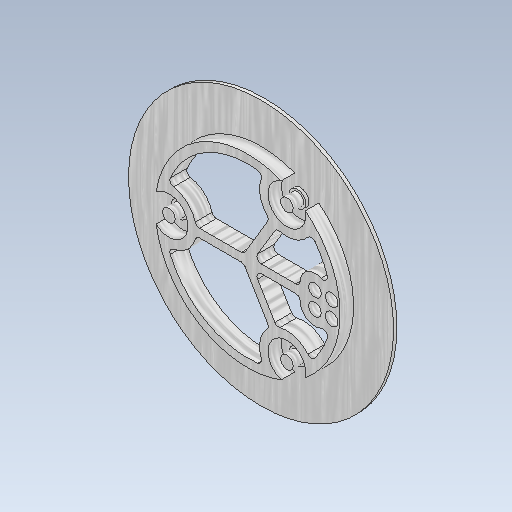
# Autodesk Inventor part: クランク4t
Saved by Autodesk Inventor 2020.2 (Build 242310000, 310)
## iProperties
Created: 2020-04-13
Part Number: クランク4t
Material: アルミニウム 7075
Document SubType Name: Modeling
Designer: aoyama
Density: 2.81 g/cm^3
Appearance: サテン - ブラシ仕上げ 重厚
Author: aoyama
Autodesk Inventor part; units mm, degrees
ref_plane "YZ Plane" through (0, 0, 0) normal (1, 0, 0) x (0, 1, 0)
ref_plane "XZ Plane" through (0, 0, 0) normal (0, 1, 0) x (-1, 0, 0)
ref_plane "XY Plane" through (0, 0, 0) normal (0, 0, 1) x (1, 0, 0)
sketch "スケッチ1" plane through (0, 0, 0) normal (0, 0, 1) x (1, 0, 0)
  circle A0 centre (-18, 0) radius 31.5
  line L0 (0, 0) -> (-18, 0) construction
  circle A1 centre (-36.7, 0) radius 1.5
  circle A2 centre (-36.7, 0) radius 4 construction
  circle A3 centre (-36.7, 0) radius 4.5
  circle A4 centre (-8.65, -16.1947) radius 4.5
  circle A5 centre (-8.65, -16.1947) radius 4 construction
  circle A6 centre (-8.65, -16.1947) radius 1.5
  circle A7 centre (-8.65, 16.1947) radius 4.5
  circle A8 centre (-8.65, 16.1947) radius 4 construction
  circle A9 centre (-8.65, 16.1947) radius 1.5
  circle A10 centre (-18, 0) radius 22
  line L1 (-36.7, 0) -> (-18, 0) construction
  circle A11 centre (-18, 0) radius 22.7 construction
  circle A12 centre (-36.7, 0) radius 2
  circle A13 centre (-8.65, -16.1947) radius 2
  circle A14 centre (-8.65, 16.1947) radius 2
  circle A15 centre (-1.9799, 1.9799) radius 2.8
  circle A16 centre (-1.9799, 1.9799) radius 1.5
  circle A17 centre (-1.9799, -1.9799) radius 1.5
  circle A18 centre (-1.9799, -1.9799) radius 2.8
  circle A19 centre (1.9799, -1.9799) radius 1.5
  circle A20 centre (1.9799, -1.9799) radius 2.8
  circle A21 centre (1.9799, 1.9799) radius 1.5
  circle A22 centre (1.9799, 1.9799) radius 2.8
  line L2 (0, 0) -> (-1.9799, 1.9799)
  point P0 (-1.5877, 1.6905)
  point P1 (-5.0591, 12.5113)
  point P2 (1.2886, 2.8639)
  point P3 (1.2886, -2.8639)
  point P4 (-5.0591, -12.5113)
  point P5 (-13.6354, -17.4628)
  point P6 (-35.3056, -4.9515)
  point P7 (-35.3056, 4.9515)
  point P8 (-13.6354, 17.4628)
  point P9 (0.5827, -2.75)
  point P10 (-4.16, 16.8432)
  point P11 (-4.16, -16.8432)
  point P12 (-10.3333, -20.4074)
  point P13 (-39.5067, -3.5642)
  point P14 (-39.5067, 3.5642)
  point P15 (-10.3333, 20.4074)
  point P16 (-0.2113, 2.75)
  point P17 (-35.9375, 1.4987)
  point P18 (-35.9375, -1.4987)
  point P19 (-7.7333, -14.785)
  point P20 (-10.3292, -16.2837)
  point P21 (-10.3292, 16.2837)
  point P22 (-7.7333, 14.785)
  point P23 (4, 0.041)
  point P24 (4, -0.041)
  point P25 (3.5801, -4.2776)
  point P26 (-4.2595, -17.1813)
  point P27 (-9.9908, -20.4903)
  point P28 (-39.7497, -3.3089)
  point P29 (-39.7497, 3.3089)
  point P30 (-9.9908, 20.4903)
  point P31 (-4.2595, 17.1813)
  point P32 (3.5801, 4.2776)
  dimension "d10" = 63
  dimension "d13" = 3
  dimension "d14" = 8
  dimension "d15" = 9
  dimension "d16" = 360
  dimension "d19" = 9.5
  dimension "d23" = 4
  dimension "d24" = 360
  dimension "d25" = 5.6
  dimension "d26" = 3
  dimension "d30" = 360
  dimension "d46" = 45
  dimension "d47" = 18
  dimension "d49" = 44
  dimension "d50" = 18.7
  dimension "d53" = 0.7
  dimension "d69" = 45.4
  constraints: 23 centre point, 15 coincident, 6 end point, 2 horizontal, 2 tangent, 44 other
  measures "d10" diameter of A0
  measures "d13" diameter of A1
  measures "d14" diameter of A2
  measures "d15" diameter of A3
  measures "d19" radial gap between concentric circles of A10 A0
  measures "d23" diameter of A12
  measures "d25" diameter of A15
  measures "d26" diameter of A16
  measures "d46" angle of L0 L2
  measures "d47" distance of L0.end point (0, 0)
  measures "d49" diameter of A10
  measures "d50" distance of A0.centre A14.centre
  measures "d53" radial gap between concentric circles of A10 A11
  measures "d69" diameter of A11
extrude "押し出し1" add sketch "スケッチ1" along normal blind 0.8 contours A0 | A3 A10 | A10 A3 | A10 A7 | A7 A10 | A10 A4 | A4 A10 | A22 A10 | A10 A20
extrude "押し出し2" add sketch "スケッチ1" along normal blind 1.5 contours A12 | A13 | A14
extrude "押し出し3" add sketch "スケッチ1" along normal blind 4 contours A1 | A3 A10 A7 A22 A15 A18 A20 A4 | A10 A22 A20 A21 A15 | A20 A18 A19 A22 A10 | A10 A20 A22 | A22 A16 A18 A15 | A15 A21 A22 A16 | A20 A17 A18 A19 | A18 A15 A17 A20 | A22 A19 A20 A21 | A18 A16 A15 A17 | A21 A20 A15 | A22 L2 A16 | A18 A22 A19 | A17 A15 A20 | A18 A16 L2 | A6 | A9 picked at (0.5491, 0.5309) picked at (0.5491, -0.5309) picked at (-0.5491, -0.5309)
sketch "スケッチ2" plane through (0, 0, 4) normal (0, 0, 1) x (1, 0, 0)
  arc A0 (-39.7497, -3.3089) -> (-39.7497, 3.3089) centre (-36.7, 0) ccw projected
  arc A1 (-39.7497, -3.3089) -> (-9.9908, -20.4903) centre (-18, 0) ccw projected
  arc A2 (-4.2595, -17.1813) -> (-9.9908, -20.4903) centre (-8.65, -16.1947) ccw projected
  arc A3 (-4.2595, -17.1813) -> (-4.2595, 17.1813) centre (-18, 0) ccw projected
  arc A4 (-9.9908, 20.4903) -> (-4.2595, 17.1813) centre (-8.65, 16.1947) ccw projected
  arc A5 (-9.9908, 20.4903) -> (-39.7497, 3.3089) centre (-18, 0) ccw projected
  circle A6 centre (1.9799, 1.9799) radius 1.5 projected
  circle A7 centre (-1.9799, -1.9799) radius 1.5 projected
  circle A8 centre (-1.9799, 1.9799) radius 1.5 projected
  circle A9 centre (1.9799, -1.9799) radius 1.5 projected
  arc A10 (-36.9155, -6.4964) -> (-36.9155, 6.4964) centre (-36.7, 0) ccw
  arc A11 (-36.9155, -6.4964) -> (-14.1683, -19.6295) centre (-18, 0) ccw
  arc A12 (-2.9162, -13.1331) -> (-14.1683, -19.6295) centre (-8.65, -16.1947) ccw
  arc A13 (-2.9162, -13.1331) -> (-2.9162, 13.1331) centre (-18, 0) ccw
  arc A14 (-14.1683, 19.6295) -> (-2.9162, 13.1331) centre (-8.65, 16.1947) ccw
  arc A15 (-14.1683, 19.6295) -> (-36.9155, 6.4964) centre (-18, 0) ccw
  circle A16 centre (-1.9799, 1.9799) radius 3.5
  circle A17 centre (-1.9799, -1.9799) radius 3.5
  line L0 (-36.7, 0) -> (0, 0) construction
  line L1 (-36.7, -1) -> (0, -1)
  line L2 (0, 1) -> (-36.7, 1)
  arc A18 (-36.7, 1) -> (-36.7, -1) centre (-36.7, 0) ccw
  arc A19 (0, -1) -> (0, 1) centre (0, 0) ccw
  line L3 (-8.65, 16.1947) -> (-18.35, 0) construction
  line L4 (-9.5079, 16.7085) -> (-19.2079, 0.5138)
  line L5 (-17.4921, -0.5138) -> (-7.7921, 15.6808)
  arc A20 (-7.7921, 15.6808) -> (-9.5079, 16.7085) centre (-8.65, 16.1947) ccw
  arc A21 (-19.2079, 0.5138) -> (-17.4921, -0.5138) centre (-18.35, 0) ccw
  line L6 (-18.35, 0) -> (-8.65, -16.1947) construction
  line L7 (-19.2079, -0.5138) -> (-9.5079, -16.7085)
  line L8 (-7.7921, -15.6808) -> (-17.4921, 0.5138)
  arc A22 (-17.4921, 0.5138) -> (-19.2079, -0.5138) centre (-18.35, 0) ccw
  arc A23 (-9.5079, -16.7085) -> (-7.7921, -15.6808) centre (-8.65, -16.1947) ccw
  circle A24 centre (-0.0604, 6.1052) radius 1.05
  circle A25 centre (-0.0604, -6.1052) radius 1.05
  point P0 (-13.5, 8.0973)
  point P1 (-13.5, -8.0973)
  point P2 (0.9336, -6.4435)
  point P3 (-0.5034, -5.1532)
  point P4 (-5.3399, -1)
  point P5 (-16.5854, -1)
  point P6 (-11.0923, -10.171)
  point P7 (-0.5034, 5.1532)
  point P8 (0.9336, 6.4435)
  point P9 (-11.0923, 10.171)
  point P10 (-16.5854, 1)
  point P11 (-5.3399, 1)
  point P12 (-12.8081, -11.1986)
  point P13 (-18.9167, -1)
  point P14 (-30.2774, -1)
  point P15 (-30.2774, 1)
  point P16 (-18.9167, 1)
  point P17 (-12.8081, 11.1986)
  dimension "d58" = 2
  dimension "d59" = 2
  dimension "d60" = 2
  dimension "d61" = 2
  dimension "d62" = 2
  dimension "d63" = 2
  dimension "d64" = 2.1
  dimension "d65" = 2.1
  constraints: 24 end point, 24 point on circle, 16 centre point, 16 tangent, 3 midpoint, 3 parallel, 5 other
  measures "d58" radial gap between concentric circles of A5 A15
  measures "d59" radial gap between concentric circles of A8 A16
  measures "d60" radial gap between concentric circles of A7 A17
  measures "d61" diameter of A19
  measures "d62" diameter of A21
  measures "d63" diameter of A23
  measures "d64" diameter of A24
  measures "d65" diameter of A25
extrude "押し出し4" cut sketch "スケッチ2" against normal blind 4 contours L1 L7 A12 A11 A10 | A10 A15 A14 L4 L2 | L8 L1 A17 A25 A13 A12 | L5 A14 A13 A24 A16 L2 | A25 | A24
fillet "フィレット1" radius 1.05 18 edges at (-30.2774, 1, 2) (-36.9155, 6.4964, 2) (-14.1683, 19.6295, 2) (-12.8081, 11.1986, 2) (-18.9167, 1, 2) (-18.9167, -1, 2) (-30.2774, -1, 2) (-36.9155, -6.4964, 2) (-14.1683, -19.6295, 2) (-12.8081, -11.1986, 2) (-2.9162, -13.1331, 2) (-11.0923, -10.171, 2) (-16.5854, -1, 2) (-5.3399, 1, 2) (-5.3399, -1, 2) (-11.0923, 10.171, 2) (-2.9162, 13.1331, 2) (-16.5854, 1, 2)
